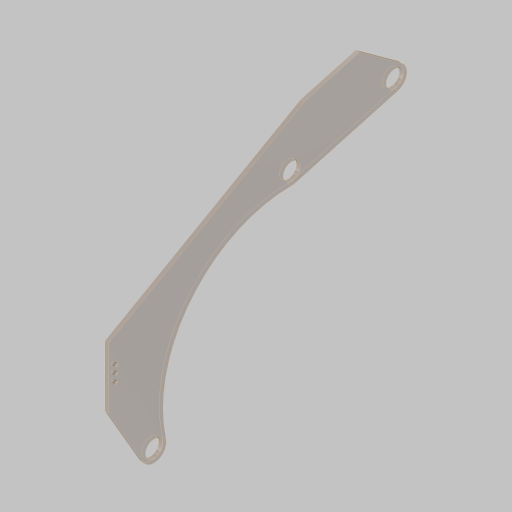
# Autodesk Inventor part: GP4-001
Saved by Autodesk Inventor 2023.5 (Build 275446000, 446)
## iProperties
Created: 2025-01-28
Part Number: GP4-001
Material: Polycarbonate, Smoke
Document SubType Name: Modeling
Designer: slick
Density: 1.2 g/cm^3
Appearance: Polycarbonate - Smoked
Author: slick
Autodesk Inventor part; units mm, degrees
ref_plane "YZ Plane" through (0, 0, 0) normal (1, 0, 0) x (0, 1, 0)
ref_plane "XZ Plane" through (0, 0, 0) normal (0, 1, 0) x (-1, 0, 0)
ref_plane "XY Plane" through (0, 0, 0) normal (0, 0, 1) x (1, 0, 0)
sketch "Sketch1" plane through (0, 0, 0) normal (1, 0, 0) x (0, 1, 0)
  circle A0 centre (0, 0) radius 203.2 construction
  circle A1 centre (234.95, 0) radius 38.1 construction
  circle A2 centre (234.95, 0) radius 31.75 construction
  circle A3 centre (-50.8, 229.3924) radius 38.1 construction
  circle A4 centre (-50.8, 229.3924) radius 31.75 construction
  circle A5 centre (282.575, -171.45) radius 38.1 construction
  circle A6 centre (282.575, -171.45) radius 31.75 construction
  line L0 (418.6545, -106.8222) -> (392.4811, 4.4408) construction
  line L1 (392.4811, 4.4408) -> (98.8705, -64.6278) construction
  line L2 (98.8705, -64.6278) -> (125.0439, -175.8908) construction
  line L3 (125.0439, -175.8908) -> (418.6545, -106.8222) construction
  line L4 (418.6545, -106.8222) -> (98.8705, -64.6278) construction
  line L5 (392.4811, 4.4408) -> (125.0439, -175.8908) construction
  line L6 (234.95, 0) -> (282.575, -171.45) construction
  point P0 (258.7625, -85.725)
  dimension "d0" = 406.4
  dimension "d1" = 76.2
  dimension "d2" = 6.35
  dimension "d4" = 114.3
  dimension "d5" = 301.625
  dimension "d6" = 50.8
  dimension "d25" = 171.45
  dimension "d26" = 47.625
  constraints: 14 end point, 7 centre point, 4 equal radius, 4 tangent, 3 midpoint, 2 coincident, 2 parallel, 1 horizontal alignment, 1 perpendicular
  measures "d0" diameter of A0
  measures "d1" diameter of A1
  measures "d2" radial gap between concentric circles of A1 A2
  measures "d4" distance of L2.end L1.end
  measures "d5" distance of L1.end L0.end
  measures "d6" horizontal distance of A3.centre point (0, 0)
  measures "d25" vertical distance of point (0, 0) L6.end
  measures "d26" horizontal distance of L6.end L6.start
sketch "Sketch4" plane through (0, 0, 0) normal (1, 0, 0) x (0, 1, 0)
  circle A0 centre (0, 0) radius 203.2 construction
  circle A1 centre (234.95, 0) radius 38.1 construction
  circle A2 centre (234.95, 0) radius 31.75 construction
  circle A3 centre (-50.8, 229.3924) radius 38.1 construction
  circle A4 centre (-50.8, 229.3924) radius 31.75 construction
  circle A5 centre (282.575, -171.45) radius 38.1 construction
  circle A6 centre (282.575, -171.45) radius 31.75 construction
  line L0 (418.6545, -106.8222) -> (392.4811, 4.4408) construction
  line L1 (392.4811, 4.4408) -> (98.8705, -64.6278) construction
  line L2 (98.8705, -64.6278) -> (125.0439, -175.8908) construction
  line L3 (125.0439, -175.8908) -> (418.6545, -106.8222) construction
  line L4 (418.6545, -106.8222) -> (98.8705, -64.6278) construction
  line L5 (392.4811, 4.4408) -> (125.0439, -175.8908) construction
  line L6 (234.95, 0) -> (282.575, -171.45) construction
  circle A7 centre (-50.8, 229.3924) radius 14.2875
  circle A8 centre (234.95, 0) radius 14.2875
  circle A9 centre (282.575, -171.45) radius 14.2875
  circle A10 centre (234.95, 0) radius 20.6375 construction
  circle A11 centre (282.575, -171.45) radius 20.6375 construction
  circle A12 centre (-50.8, 229.3924) radius 20.6375 construction
  line L7 (262.6904, -176.9735) -> (215.0654, -5.5235)
  line L8 (350.3831, -113.0583) -> (324.89, -21.2832)
  line L9 (350.3831, -113.0583) -> (299.2852, -183.561)
  line L10 (324.89, -21.2832) -> (139.7, 304.8)
  line L11 (139.7, 304.8) -> (38.1, 304.8)
  line L12 (38.1, 304.8) -> (-61.1526, 247.2454)
  arc A13 (214.3125, 0) -> (-46.3378, 209.243) centre (0, 0) ccw
  arc A14 (214.3125, 0) -> (215.0654, -5.5235) centre (234.95, 0) ccw
  arc A15 (262.6904, -176.9735) -> (299.2852, -183.561) centre (282.575, -171.45) ccw
  line L13 (405.5678, -51.1907) -> (111.9572, -120.2593) construction
  arc A16 (-61.1526, 247.2454) -> (-46.3378, 209.243) centre (-50.8, 229.3924) ccw
  point P0 (258.7625, -85.725)
  point P1 (337.6366, -67.1708)
  dimension "d27" = 28.575
  dimension "d28" = 6.35
  dimension "d29" = 6.35
  dimension "d30" = 6.35
  dimension "d31" = 101.6
  dimension "d32" = 304.8
  dimension "d33" = 101.6
  dimension "d34" = 38.1
  dimension "d35" = 95.25
  constraints: 15 end point, 15 point on circle, 10 centre point, 7 coincident, 5 tangent, 3 equal radius, 3 midpoint, 1 horizontal, 1 parallel, 1 point on line
  measures "d27" diameter of A7
  measures "d28" radial gap between concentric circles of A8 A10
  measures "d29" radial gap between concentric circles of A9 A11
  measures "d30" radial gap between concentric circles of A7 A12
  measures "d31" distance between parallel lines of L7 L8
  measures "d32" distance from line of point (0, 0) L11
  measures "d33" distance of L10.end L11.end
  measures "d34" horizontal distance of point (0, 0) L11.end
  measures "d35" distance of L8.start L8.end
extrude "Extrusion2" add sketch "Sketch4" along normal blind 6.35
sketch "Sketch5" plane through (6.35, 0, 0) normal (1, 0, 0) x (0, 0, -1)
  line L0 (-304.8, 139.7) -> (-304.8, 38.1) projected
  point P0 (0, 0)
  point P1 (-292.1, 101.6)
  point P2 (-292.1, 88.9)
  point P3 (-292.1, 76.2)
  point P4 (-304.8, 88.9)
  dimension "d38" = 12.7
  dimension "d39" = 12.7
  dimension "d40" = 12.7
  constraints: 2 vertical alignment, 1 horizontal alignment, 1 midpoint
  measures "d38" distance of point (-292.1, 88.9) point (-292.1, 101.6)
  measures "d39" distance from line of L0 point (-292.1, 101.6)
  measures "d40" distance of point (-292.1, 76.2) point (-292.1, 88.9)
hole "Hole2" at (6.35, 101.6, 292.1) at (6.35, 88.9, 292.1) at (6.35, 76.2, 292.1) direction (-1, 0, 0) diameter 5.1054 end through all clearance for "Flat Head Machine Screw (82)" size "#10" standard "Ansi Unified Screw Threads"
body "Solid2"
